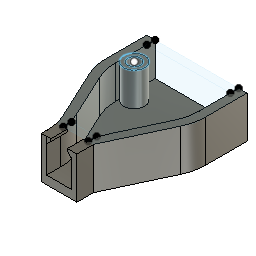
Heat Bed Cable Relief (Autodesk Fusion 360 design; units mm, degrees)
Autodesk Fusion 360 part; units mm, degrees
sketch "Sketch1" plane through (0, 0, 0) normal (0, 0, 1) x (1, 0, 0)
  line L0 (10, -10) -> (-10, -10) construction
  line L1 (-10, -10) -> (-10, 10) construction
  line L2 (-10, 10) -> (10, 10) construction
  line L3 (10, 10) -> (10, -10) construction
  line L4 (10, -10) -> (-10, 10) construction
  line L5 (-10, -10) -> (10, 10) construction
  line L6 (0, 0) -> (0, -44.6204) construction
  line L7 (3, 5) -> (-3, 5) construction
  line L8 (-3, 5) -> (-3, -25) construction
  line L9 (-3, -25) -> (3, -25) construction
  line L10 (3, -25) -> (3, 5) construction
  line L11 (3, 5) -> (-3, -25) construction
  line L12 (-3, 5) -> (3, -25) construction
  line L13 (-3, -25) -> (3, -25)
  line L14 (10, -10) -> (3, -25)
  line L15 (-3, -25) -> (-10, -10)
  line L16 (-10, 0) -> (-10, -10)
  line L17 (10, -10) -> (10, 0)
  line L18 (-10, 0) -> (10, 0)
  line L19 (-4.2737, -27) -> (4.2737, -27)
  line L20 (12, -10.4437) -> (4.2737, -27)
  line L21 (12, -10.4437) -> (12, 2)
  line L22 (-12, 2) -> (12, 2)
  line L23 (-12, 2) -> (-12, -10.4437)
  line L24 (-4.2737, -27) -> (-12, -10.4437)
  point P0 (0, -10)
  dimension "d1" = 20
  dimension "d2" = 20
  dimension "d3" = 6
  dimension "d4" = 30
  dimension "d5" = -2
  constraint perpendicular L0 L1
  constraint parallel L0 L2
  constraint parallel L1 L3
  constraint horizontal L0
  constraint coincident L4 L6.start
  constraint coincident L5 L6.start
  constraint coincident L6.start origin
  constraint perpendicular L0 L6
  constraint perpendicular L7 L8
  constraint parallel L7 L9
  constraint parallel L8 L10
  constraint horizontal L7
  constraint coincident L11 P0
  constraint coincident L12 P0
  constraint midpoint L0 P0
  constraint midpoint L1 L16.start
  constraint midpoint L3 L17.end
  measures "d1" distance of L1.end L2.end
  measures "d2" distance of L0.end L1.end
  measures "d3" distance of L8.end L9.end
  measures "d4" distance of L7.end L8.end
extrude "Extrude1" add sketch "Sketch1" along normal blind 8
sketch "Sketch2" plane through (0, 0, 0) normal (0, 0, -1) x (1, 0, 0)
  line L0 (-3, 25) -> (3, 25)
  line L1 (3, 25) -> (10, 10)
  line L2 (10, 10) -> (10, 0)
  line L3 (10, 0) -> (-10, 0)
  line L4 (-10, 0) -> (-10, 10)
  line L5 (-10, 10) -> (-3, 25)
  line L6 (12, -2) -> (12, 10.4437)
  line L7 (12, 10.4437) -> (4.2737, 27)
  line L8 (4.2737, 27) -> (-4.2737, 27)
  line L9 (-4.2737, 27) -> (-12, 10.4437)
  line L10 (-12, 10.4437) -> (-12, -2)
  line L11 (-12, -2) -> (12, -2)
extrude "Extrude2" add sketch "Sketch2" along normal blind 2 contours L0 L1 L2 L3 L4 L5 | L6 L7 L8 L9 L10 L11
sketch "Sketch3" plane through (0, 0, 8) normal (0, 0, 1) x (-1, 0, 0)
  line L0 (-3, 25) -> (3, 25)
  line L1 (3, 25) -> (10, 10)
  line L2 (10, 10) -> (10, 0)
  line L3 (10, 0) -> (-10, 0)
  line L4 (-10, 0) -> (-10, 10)
  line L5 (-10, 10) -> (-3, 25)
  line L6 (-12, 10.4437) -> (-12, -2)
  line L7 (-12, -2) -> (12, -2)
  line L8 (12, -2) -> (12, 10.4437)
  line L9 (12, 10.4437) -> (4.2737, 27)
  line L10 (4.2737, 27) -> (-4.2737, 27)
  line L11 (-4.2737, 27) -> (-12, 10.4437)
  circle A0 centre (8, 5) radius 1.5
  circle A1 centre (8, 5) radius 2.5
  line L12 (10, 0) -> (10, -2)
  line L13 (-10, 0) -> (-10, -2)
  line L14 (-3, 25) -> (-3, 27)
  line L15 (3, 25) -> (3, 27)
  dimension "d10" = 3
  dimension "d11" = 5
  dimension "d12" = 4
  constraint concentric A0 A1
  constraint coincident L2.end L3.start
  constraint coincident L7 L12.end
  constraint perpendicular L7 L12
  constraint coincident L3.end L4.start
  constraint coincident L7 L13.end
  constraint perpendicular L7 L13
  constraint coincident L0.start L5.end
  constraint coincident L10 L14.end
  constraint perpendicular L10 L14
  constraint coincident L0.end L1.start
  constraint coincident L10 L15.end
  constraint perpendicular L10 L15
  measures "d10" diameter of A0
  measures "d11" diameter of A1
  measures "d12" distance of L8 A0.centre
extrude "Extrude4" cut sketch "Sketch3" against normal blind 8 contours L0 L10 L14 L15 | L3 L7 L12 L13
extrude "Extrude3" add sketch "Sketch3" against normal up to surface (8 mm away) contours L2 A1 picked at (9.8333, 5)
extrude "Extrude5" add 1 faces at (-1, -27, -1.3333) along direction (0, -1, 0) blind 4
fillet "Fillet1" chord length 5 7 edges at (-10, -10, 4) (-3, -25, 4) (-12, -10.4437, 3) (-4.2737, -27, 3) (3, -25, 4) (10, -10, 4) (12, -10.4437, 3)
sketch "Sketch4" plane through (0, 0, 8) normal (0, 0, 1) x (-1, 0, 0)
  spline S0 degree 3 poles (-12, 7.8829) (-12, 8.7237) (-11.9081, 9.5621) (-11.5439, 11.2038) (-11.2727, 12.0023) (-10.9171, 12.7642) knots 0 0 0 0 0.252247 0.252247 0.504494 0.504494 0.504494 0.504494
  line L0 (-12, 7.8829) -> (-12, -2)
  line L1 (-12, -2) -> (-10, -2)
  line L2 (-10, -2) -> (-10, 7.4392)
  spline S1 degree 3 poles (-8.9171, 12.3205) (-9.2727, 11.5586) (-9.5439, 10.7601) (-9.9081, 9.1184) (-10, 8.28) (-10, 7.4392) knots 0 0 0 0 0.252247 0.252247 0.504494 0.504494 0.504494 0.504494
  line L3 (-8.9171, 12.3205) -> (-4.0829, 22.6795)
  spline S2 degree 3 poles (-3, 27.5608) (-3, 26.72) (-3.0919, 25.8816) (-3.4561, 24.2399) (-3.7273, 23.4414) (-4.0829, 22.6795) knots 0 0 0 0 0.252247 0.252247 0.504494 0.504494 0.504494 0.504494
  line L4 (-3, 27.5608) -> (-3, 31)
  line L5 (-3, 31) -> (-4.2737, 31)
  line L6 (-4.2737, 31) -> (-4.2737, 27)
  line L7 (-4.2737, 27) -> (-10.9171, 12.7642)
  line L8 (-3, 31) -> (-2, 31)
  line L9 (-2, 31) -> (-2, 27)
  line L10 (-2, 27) -> (-3, 27)
  line L11 (-3, 27) -> (-3, 31)
  line L12 (3.0196, 30.9519) -> (2.0196, 30.9519)
  line L13 (2.0196, 30.9519) -> (2.0196, 27)
  line L14 (2.0196, 27) -> (3.0196, 27)
  line L15 (3.0196, 27) -> (3.0196, 30.9519)
  dimension "d20" = 1
  dimension "d21" = 1
  constraint horizontal L8
  constraint vertical L9
  constraint horizontal L10
  constraint vertical L11
  constraint coincident L4.end L5.start
  constraint horizontal L12
  constraint vertical L13
  constraint horizontal L14
  constraint vertical L15
  measures "d20" distance of L4.end L8.end
  measures "d21" distance of L12.start L12.end
extrude "Extrude6" add sketch "Sketch4" against normal blind 1.5 contours L4 L8 L9 L10 L11 | L12 L13 L14 L15
chamfer "Chamfer1" distance 0.9 angle 45 2 edges at (-2.0196, -28.976, 6.5) (2, -29, 6.5)
